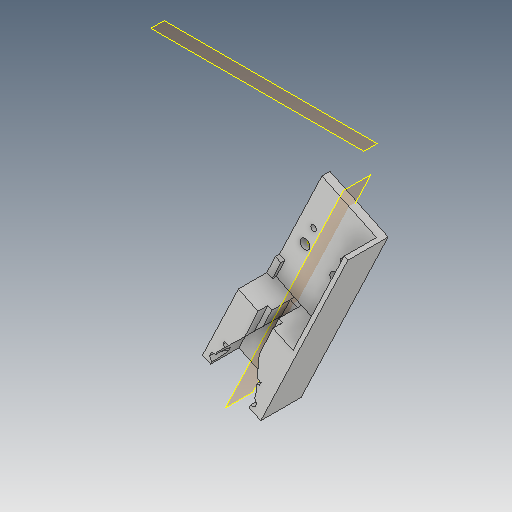
# Autodesk Inventor part: 30_CUBE_openSIM_Laser_Telescope_Mount
Saved by Autodesk Inventor 2019 (Build 230136000, 136)
## iProperties
Created: 2020-03-02
Part Number: 30_CUBE_openSIM_Laser_Telescope_Mount
Material: Generic
Document SubType Name: Modeling
Designer: diederichbenedict
Density: 1 g/cm^3
Appearance: Default
Author: diederichbenedict
Autodesk Inventor part; units mm, degrees
ref_plane "YZ Plane" through (0, 0, 0) normal (1, 0, 0) x (0, 1, 0)
ref_plane "XZ Plane" through (0, 0, 0) normal (0, 1, 0) x (-1, 0, 0)
ref_plane "Work Plane1" through (0, 0, 1.5) normal (0, 0, 1) x (1, 0, 0)
sketch "Sketch1" plane through (0, 0, 1.5) normal (0, 0, 1) x (1, 0, 0)
  line L0 (8.75354, 57.756452) -> (7.809034, 57.756452) construction
  line L1 (-24.776894, -15.05709) -> (8.75354, 57.756452) construction
  line L2 (-24.776894, -52.66184) -> (-24.776894, -15.05709) construction
  line L3 (-18.707308, -55.556884) -> (-24.776894, -52.66184) construction
  line L4 (-18.707308, -40.563421) -> (-18.707308, -55.556884) construction
  line L5 (0.391621, -40.563421) -> (-18.707308, -40.563421) construction
  line L6 (23.692692, 8.28829) -> (0.391621, -40.563421) construction
  line L7 (23.692692, 53.178978) -> (23.692692, 8.28829) construction
  line L8 (8.974225, 60.199326) -> (23.692692, 53.178978) construction
  line L9 (7.809034, 57.756452) -> (8.974225, 60.199326) construction
  circle A0 centre (-21.307308, -37.886297) radius 1.6 construction
  circle A1 centre (-21.307308, -27.886297) radius 1.6 construction
  line L10 (11.632256, -10.582296) -> (32.395806, 32.949392)
  line L11 (-15.355044, 2.289986) -> (5.408506, 45.821674)
  line L12 (5.408506, 45.821674) -> (32.395806, 32.949392)
  line L13 (32.395806, 32.949392) -> (-10.655303, -57.309136)
  line L14 (-10.655303, -57.309136) -> (-37.642603, -44.436855)
  line L15 (-37.642603, -44.436855) -> (5.408506, 45.821674)
  circle A2 centre (11.737087, 5.432666) radius 3
  circle A3 centre (-13.983408, -29.560487) radius 3
  circle A4 centre (-2.975053, 12.449997) radius 3
  point P0 (0, 0)
  dimension "d1" = 100
  constraints: 8 end point, 2 parallel, 2 perpendicular
  measures "d1" distance of L10.end L13.end
ref_plane "Work Plane2" through (4.456703, -9.721274, 3.970957) normal (0, 0, -1) x (0.4305111, 0.9025853, 0)
extrude "Extrusion1" add sketch "Sketch1" along normal up to surface (2.470957 mm away) contours L13 L14 L15 L11 L12 L10 | A2 | A3 | A4
sketch "Sketch2" plane through (-10.655303, -57.309136, 3.970957) normal (0, 0, 1) x (0.9025853, -0.4305111, 0)
  line L0 (0, 0) -> (0, 100)
  line L1 (0, 100) -> (-29.9, 100)
  line L2 (-29.9, 100) -> (-29.9, 0)
  line L3 (-29.9, 0) -> (0, 0)
  line L4 (-21.95, 51.77) -> (-27.9, 51.77)
  line L5 (-2, 51.77) -> (-7.95, 51.77)
  line L6 (-19.05, 34.77) -> (-10.85, 34.77)
  arc A0 (-27.45, 2.77) -> (-2.45, 2.77) centre (-14.95, 20.30125) ccw construction
  arc A1 (-2.45, 4.77) -> (-27.45, 4.77) centre (-14.95, -12.76125) ccw construction
  line L7 (-27.45, 2.77) -> (-27.45, 4.77) construction
  line L8 (-2.45, 2.77) -> (-2.45, 4.77) construction
  line L9 (-29.9, 0) -> (0, 0)
  line L10 (-25.477276, 0) -> (-25.477276, 7.745132)
  line L11 (-25.477276, 7.745132) -> (-16.899837, 31.078166)
  line L12 (-16.899837, 31.078166) -> (-16.899837, 41.065184)
  line L13 (-16.899837, 41.065184) -> (-29.9, 41.24513)
  line L14 (-29.9, 100) -> (-29.9, 0)
  line L15 (-29.9, 0) -> (-29.9, 41.24513)
  line L16 (-14.95, 0) -> (-14.95, 40.435372) construction
  line L17 (-2.45, 2.77) -> (-2.45, 4.77) construction
  line L18 (-4.422724, 0) -> (-4.422724, 7.745132)
  line L19 (-4.422724, 7.745132) -> (-13.000163, 31.078166)
  line L20 (-13.000163, 31.078166) -> (-13.000163, 41.065184)
  line L21 (-13.000163, 41.065184) -> (0, 41.24513)
  line L22 (0, 0) -> (0, 41.24513)
  line L23 (0, 0) -> (0, 100) construction
  line L24 (0, 41.24513) -> (0, 0) construction
  line L25 (0, 0) -> (-4.422724, 0) construction
  point P0 (-15.054899, 56.31361)
  constraints: 32 end point, 5 symmetric about line, 4 point on circle, 3 vertical, 2 centre point, 2 collinear, 2 perpendicular, 2 point on line, 1 midpoint, 1 parallel, 8 other
extrude "Extrusion2" add sketch "Sketch2" along normal blind 16 contours L3 L2 L13 L12 L11 L10
ref_plane "Work Plane3" through (-24.148953, -50.872995, 3.970957) normal (0.9025853, -0.4305111, 0) x (0, 0, -1)
mirror "Mirror1" about plane through (-24.148953, -50.872995, 3.970957) normal (0.9025853, -0.4305111, 0) of "Extrusion2"
sketch "Sketch3" plane through (-4.710042, -14.647591, 19.970957) normal (0.4179776, 0.9084573, 0) x (0.9084573, -0.4179776, 0)
  ellipse E0 centre (-1.967577, -0.95) end of major axis (-1.967577, 1.897221) minor radius 2.846948 construction
  line L0 (2.132031, -4.8) -> (2.132031, 2.9) construction
  line L1 (2.132031, 2.9) -> (-6.067184, 2.9) construction
  line L2 (-6.067184, 2.9) -> (-6.067184, -4.8) construction
  line L3 (-6.067184, -4.8) -> (2.132031, -4.8) construction
  line L4 (2.132031, -4.8) -> (2.132031, 2.9)
  line L5 (2.132031, 2.9) -> (-6.067184, 2.9)
  line L6 (-6.067184, 2.9) -> (-6.067184, -4.8)
  line L7 (-6.067184, -4.8) -> (2.132031, -4.8)
  line L8 (2.132031, 2.9) -> (-6.067184, 2.9)
  line L9 (-6.067184, 2.9) -> (-6.067184, 3.9)
  line L10 (-6.067184, 3.9) -> (2.132031, 3.9)
  line L11 (2.132031, 3.9) -> (2.132031, 2.9)
  ellipse E1 centre (-2.037491, 0.97324) end of major axis (-2.037491, 3.820462) minor radius 2.846948
  line L12 (2.062116, -2.87676) -> (2.062116, 4.82324)
  line L13 (-6.137098, -2.87676) -> (2.062116, -2.87676)
  line L14 (-6.137098, 4.82324) -> (-6.137098, -2.87676)
  line L15 (2.062116, 4.82324) -> (-6.137098, 4.82324)
  point P0 (-1.843493, 19.970957)
  dimension "d6" = 0
  dimension "d40" = 1
  constraints: 16 end point, 2 parallel, 1 horizontal, 1 perpendicular, 5 other
  measures "d6" distance between parallel lines of L3 L7
  measures "d40" distance of L8.end L9.end
extrude "Extrusion3" cut sketch "Sketch3" along normal through all both and the other way through all contours L5 L12 L10 L11 | L12 L13 L6 L5 E1 | L5 E1 L9 L10 L12 | L13 L14 L15 L12 L10 L9 L6 | E1 L5 | L5 E1
sketch "Sketch4" plane through (-24.148953, -50.872995, 3.970957) normal (0.9025853, -0.4305111, 0) x (0, 0, -1)
  arc A0 (-27.45, 2.77) -> (-2.45, 2.77) centre (-14.95, 20.30125) ccw
  line L0 (-27.45, 2.77) -> (-27.45, 4.77)
  arc A1 (-2.45, 4.77) -> (-27.45, 4.77) centre (-14.95, -12.76125) ccw
  arc A2 (-2.475103, 4.91042) -> (-27.55, 4.82144) centre (-14.95, -12.76125) ccw
  line L1 (-27.55, 4.82144) -> (-27.55, 2.71856)
  arc A3 (-27.55, 2.71856) -> (-2.475103, 2.62958) centre (-14.95, 20.30125) ccw
  line L2 (-15.02676, 8.869864) -> (-15.02676, -1.329864)
  point P0 (3.970957, 56.31361)
  dimension "d9" = 0.1
  constraints: 10 point on circle, 6 end point, 4 centre point, 1 vertical, 10 other
  measures "d9" radial gap between concentric circles of A1 A2
revolve "Revolution1" cut sketch "Sketch4" angle 360 about axis through (-20.330379, -42.867187, 18.997716) along (-0.4305111, -0.9025853, 0)
sketch "Sketch5" plane through (0, 0, 1.5) normal (0, 0, -1) x (-1, 0, 0)
  circle A0 centre (-11.737087, 5.432666) radius 3 construction
  circle A1 centre (2.975053, 12.449997) radius 3 construction
  point P0 (0, 0)
sketch "Sketch6" plane through (0, 0, 1.5) normal (0, 0, -1) x (-1, 0, 0)
  circle A0 centre (13.983408, -29.560487) radius 1.4
  circle A1 centre (-11.737087, 5.432666) radius 1.4
  circle A2 centre (2.975053, 12.449997) radius 1.4
  arc A3 (-15.34796, 15.674263) -> (-14.660489, 14.23295) centre (-16.042198, 14.458519) ccw
  ellipse E0 centre (-0.984271, 21.640781) end of major axis (-0.381556, 20.377162) minor radius 1.212436 (-0.021072, 22.388567) -> (0.203028, 21.918731) ccw
  arc A4 (-0.200517, 22.302976) -> (0.023583, 21.83314) centre (-1.330058, 21.47585) ccw
  circle A5 centre (13.983408, -29.560487) radius 2.45
  circle A6 centre (-11.737087, 5.432666) radius 2.45
  circle A7 centre (2.975053, 12.449997) radius 2.45
  circle A8 centre (-16.042198, 14.458519) radius 1.45
  circle A9 centre (-1.330058, 21.47585) radius 1.45
  point P0 (0, 0)
  dimension "d11" = 4.9
  dimension "d12" = 4.9
  dimension "d13" = 4.9
  dimension "d14" = 2.9
  dimension "d15" = 2.9
  constraints: 5 centre point, 5 coincident, 1 other
  measures "d11" diameter of A5
  measures "d12" diameter of A6
  measures "d13" diameter of A7
  measures "d14" diameter of A8
  measures "d15" diameter of A9
sketch "Sketch7" plane through (5.408506, 45.821674, 3.970957) normal (0, 0, 1) x (0.9025853, -0.4305111, 0)
  line L0 (25.477276, -100) -> (25.477276, -92.254868)
  line L1 (25.477276, -92.254868) -> (16.899837, -68.921834)
  line L2 (16.899837, -68.921834) -> (16.899837, -58.934816)
  line L3 (16.899837, -58.934816) -> (29.9, -58.75487)
  line L4 (29.9, -58.75487) -> (29.9, 0)
  line L5 (29.9, 0) -> (0, 0)
  line L6 (0, 0) -> (0, -58.75487)
  line L7 (0, -58.75487) -> (13.000163, -58.934816)
  line L8 (13.000163, -58.934816) -> (13.000163, -68.921834)
  line L9 (13.000163, -68.921834) -> (4.422724, -92.254868)
  line L10 (4.422724, -92.254868) -> (4.422724, -100)
  line L11 (4.422724, -100) -> (25.477276, -100)
  line L12 (0, -58.75487) -> (3, -58.75487)
  line L13 (3, -58.75487) -> (3, -48.75487)
  line L14 (3, -48.75487) -> (0, -48.75487)
  line L15 (0, -48.75487) -> (0, -58.75487)
  line L16 (16.899837, -58.934816) -> (29.9, -58.75487)
  line L17 (29.9, -58.75487) -> (26.9, -58.75487)
  line L18 (26.9, -58.75487) -> (26.9, -48.75487)
  line L19 (26.9, -48.75487) -> (29.9, -48.75487)
  line L20 (29.9, -48.75487) -> (29.9, -58.75487)
  line L21 (13.000163, -58.934816) -> (13.000163, -68.921834)
  line L22 (13.000163, -58.934816) -> (16.899837, -58.934816)
  point P0 (14.845101, -43.68639)
  point P1 (2, -48.23)
  dimension "d18" = 3
  dimension "d19" = 10
  dimension "d20" = 3
  dimension "d21" = 10
  constraints: 18 end point, 4 parallel, 3 perpendicular, 2 horizontal, 1 other
  measures "d18" distance of L14.end L13.end
  measures "d19" distance of L13.end L12.end
  measures "d20" distance of L18.end L19.end
  measures "d21" distance of L17.end L18.end
extrude "Extrusion5" add sketch "Sketch7" along normal blind 2 contours L11 L10 L9 L8 L22 L2 L1 L0 | L17 L18 L19 L4 | L6 L14 L13 L12
extrude "Extrusion6" cut sketch "Sketch6" against normal blind 3 contours A0 | A1 | A2 | A9 E0 | E0 A4 A9 | E0 A4 | A5 | A6 | A7 | A8
sketch "Sketch8" plane through (32.395806, 32.949392, 3.970957) normal (0.9025853, -0.4305111, 0) x (0, 0, -1)
  line L0 (2.470957, -100) -> (-16, -100)
  line L1 (2.470957, -100) -> (2.470957, 0)
  line L2 (2.470957, 0) -> (0, 0)
  line L3 (0, -48.75487) -> (0, 0)
  line L4 (0, -48.75487) -> (-2, -48.75487)
  line L5 (-2, -58.75487) -> (-2, -48.75487)
  line L6 (0, -58.75487) -> (-2, -58.75487)
  line L7 (-2, -58.75487) -> (-16, -58.75487)
  line L8 (-16, -58.75487) -> (-16, -100)
  line L9 (-16, -100) -> (2.470957, -100)
  line L10 (2.470957, -100) -> (2.470957, 0)
  line L11 (2.470957, 0) -> (-16, 0)
  line L12 (-16, 0) -> (-16, -100)
  point P0 (3.970957, -43.68639)
  constraints: 8 end point, 2 parallel, 1 horizontal, 1 perpendicular
extrude "Extrusion7" add sketch "Sketch8" along normal blind 2
sketch "Sketch9" plane through (0, 0, 1.5) normal (0, 0, -1) x (-1, 0, 0)
  circle A0 centre (-11.737087, 5.432666) radius 2.45
  circle A1 centre (-1.330058, 21.47585) radius 1.45
  circle A2 centre (-16.042198, 14.458519) radius 1.45
  circle A3 centre (13.983408, -29.560487) radius 2.45
  circle A4 centre (2.975053, 12.449997) radius 2.45
  line L0 (-34.200977, 32.08837) -> (-5.408506, 45.821674)
  line L1 (8.850133, -58.170159) -> (-34.200977, 32.08837)
  line L2 (37.642603, -44.436855) -> (8.850133, -58.170159)
  line L3 (-5.408506, 45.821674) -> (37.642603, -44.436855)
  point P0 (0, 0)
extrude "Extrusion8" add sketch "Sketch9" along normal blind 1.5
ref_plane "Work Plane4" through (-74.107308, 67.113703, 4) normal (0, 1, 0) x (1, 0, 0)
sketch "Sketch10" plane through (-74.107308, 67.113703, 4) normal (0, 1, 0) x (1, 0, 0)
  circle A0 centre (47.977855, 3.12324) radius 3
  circle A1 centre (47.977855, 3.12324) radius 4.301236
  point P0 (74.107308, 4)
  constraints: 1 centre point
extrude "Extrusion9" cut sketch "Sketch10" against normal through all contours A0 | A1
sketch "Sketch11" plane through (0, 0, 0) normal (0, 0, -1) x (-1, 0, 0)
  circle A0 centre (-1.330058, 21.47585) radius 1.45
  circle A1 centre (-16.042198, 14.458519) radius 1.45
  point P0 (0, 0)
hole "Hole1" at (16.042198, 14.458519, 0) at (1.330058, 21.47585, 0) direction (0, 0, 1) diameter 2.9 end through all counterbore diameter 6 counterbore depth 2
sketch "Sketch12" plane through (-24.148953, -50.872995, 3.970957) normal (0.9025853, -0.4305111, 0) x (0, 0, -1)
  line L0 (-25.02676, 14.71856) -> (-5.02676, 14.71856)
  line L1 (-25.02676, 14.71856) -> (-25.02676, 13.31856)
  arc A0 (-25.02676, 13.31856) -> (-15.093782, 10.018425) centre (-15.093782, 26.616977) ccw
  line L2 (-5.02676, 14.81856) -> (-25.12676, 14.81856)
  line L3 (-25.12676, 14.81856) -> (-25.12676, 13.268531)
  arc A1 (-25.12676, 13.268531) -> (-15.093782, 9.918425) centre (-15.093782, 26.616977) ccw
  line L4 (-15.093782, 9.918425) -> (-15.093782, 14.81856)
  line L5 (-15.093782, 9.918425) -> (-10.193647, 9.918425) construction
  point P0 (3.970957, 56.31361)
  dimension "d41" = 0.1
  dimension "d42" = 90
  constraints: 10 end point, 4 point on circle, 2 centre point, 2 point on line, 1 horizontal, 1 perpendicular, 1 vertical, 6 other
  measures "d41" distance between parallel lines of L0 L2
  measures "d42" angle of L5 L4
revolve "Revolution2" cut sketch "Sketch12" angle 360 about axis through (-19.878961, -41.920771, 19.064739) along (0.4305111, 0.9025853, 0)
body "Solid1"
